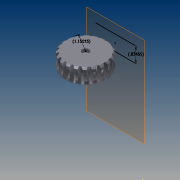
# Autodesk Inventor part: Worm Gear
Saved by Autodesk Inventor 2015 SP1 (Build 190203100, 203)
## iProperties
Created: 2015-04-26
Part Number: Worm Gear
Material: ABS Plastic
Document SubType Name: Modeling
Designer: Trevor
Categories: <?xml version="1.0" encoding="UTF-16"?> <MemberInstance><Categories><FamilyTemplate><FamilyTemplateParameter ValueType="xs:double" Id="1" ObjectReferenceKey="da_z" ObjectType="kUserParameterObject"/><FamilyTemplateParameter ValueType="xs:double" Id="2" ObjectReferenceKey="da_b" ObjectType="kUserParameterObject"/><FamilyTemplateParameter ValueType="xs:double" Id="3" ObjectReferenceKey="da_beta" ObjectType="kUserParameterObject"/><FamilyTemplateParameter ValueType="xs:double" Id="4" ObjectReferenceKey="da_m" ObjectType="kUserParameterObject"/><FamilyTemplateParameter ValueType="xs:double" Id="5" ObjectReferenceKey="da_alpha" ObjectType="kUserParameterObject"/><FamilyTemplateParameter ValueType="xs:double" Id="6" ObjectReferenceKey="da_da" ObjectType="kUserParameterObject"/><FamilyTemplateParameter ValueType="xs:double" Id="7" ObjectReferenceKey="da_aw" ObjectType="kUserParameterObject"/><FamilyTemplateParameter ValueType="xs:double" Id="8" ObjectReferenceKey="da_px" ObjectType="kUserParameterObject"/><FamilyTemplateParameter ValueType="xs:double" Id="9" ObjectReferenceKey="da_d" ObjectType="kUserParameterObject"/><FamilyTemplateParameter ValueType="xs:double" Id="10" ObjectReferenceKey="da_dae" ObjectType="kUserParameterObject"/><FamilyTemplateParameter ValueType="xs:double" Id="11" ObjectReferenceKey="da_fi" ObjectType="kUserParameterObject"/><FamilyTemplateParameter ValueType="xs:string" Id="12" ObjectReferenceKey="EAIAABAAAAAWFwAAAAAAAIAAAAAAAAAA" ObjectType="83910656" SubObjectId="SurfaceGeometry"/></FamilyTemplate><ParamToTemplateMap><ParamToTemplate CategoryParameter="//CategoryParameter[@InternalName='046C89C9-8512-4d59-83FE-43B91F4F132A']" TemplateParameter="1"/><ParamToTemplate CategoryParameter="//CategoryParameter[@InternalName='2552DF32-E462-4b46-AEBF-C6C7768E72AC']" TemplateParameter="2"/><ParamToTemplate CategoryParameter="//CategoryParameter[@InternalName='C9EE641D-15FC-4fae-A226-E94C4372FDD7']" TemplateParameter="3"/><ParamToTemplate><ParamToTemplate CategoryParameter="//CategoryParameter[@InternalName='00B6519A-459B-49c7-AD84-2E56D39A5744']" ConstantValue="0.000000"/></ParamToTemplate><ParamToTemplate><ParamToTemplate CategoryParameter="//CategoryParameter[@InternalName='04B31F0E-C7A6-4894-AA32-9629BEFACF47']" ConstantValue="1.000000"/></ParamToTemplate><ParamToTemplate><ParamToTemplate CategoryParameter="//CategoryParameter[@InternalName='43CBEC2E-7847-49e7-A936-2F7889FCB2D9']" ConstantValue="0.200000"/></ParamToTemplate><ParamToTemplate><ParamToTemplate CategoryParameter="//CategoryParameter[@InternalName='B1EFC894-105D-4ebd-86BF-FA20ED196853']" ConstantValue="0.300000"/></ParamToTemplate><ParamToTemplate><ParamToTemplate CategoryParameter="//CategoryParameter[@InternalName='51175063-3D10-4879-93E8-6246FE8B403D']" ConstantValue="2060110000.000000"/></ParamToTemplate><ParamToTemplate><ParamToTemplate CategoryParameter="//CategoryParameter[@InternalName='A3A52E27-4454-46a9-B0BD-C932399B70AF']" ConstantValue="0.300000"/></ParamToTemplate><ParamToTemplate CategoryParameter="//CategoryParameter[@InternalName='91B76062-C214-41d9-B1B9-14D2AB99603D']" TemplateParameter="4"/><ParamToTemplate CategoryParameter="//CategoryParameter[@InternalName='2D373A89-B862-43d6-8D0B-0CBF12AB9F6C']" TemplateParameter="5"/><ParamToTemplate CategoryParameter="//CategoryParameter[@InternalName='37777632-D6A2-4fac-9D53-DB8ACD95C989']" TemplateParameter="6"/><ParamToTemplate CategoryParameter="//CategoryParameter[@InternalName='FD1017F1-B727-4f7e-9707-0F86F1FF9423']" TemplateParameter="7"/><ParamToTemplate CategoryParameter="//CategoryParameter[@InternalName='3BF567DA-17EF-48d8-80EA-D119B07F6463']" TemplateParameter="8"/><ParamToTemplate CategoryParameter="//CategoryParameter[@InternalName='BF5A1E7E-5373-4a22-AAD3-F583781FCF3C']" TemplateParameter="9"/><ParamToTemplate CategoryParameter="//CategoryParameter[@InternalName='2A200944-5A8C-41ca-B96E-8520D2E510F1']" TemplateParameter="10"/><ParamToTemplate CategoryParameter="//CategoryParameter[@InternalName='E77AC4FD-7B43-4566-B0ED-7CA70B976BC8']" TemplateParameter="11"/><ParamToTemplate><ParamToTemplate CategoryParameter="//CategoryParameter[@InternalName='D4F72237-D604-435a-AD0B-F738B7463A00']" ConstantValue="110.000000"/></ParamToTemplate><ParamToTemplate><ParamToTemplate CategoryParameter="//CategoryParameter[@InternalName='9E1B4470-B2D3-4ff1-B813-535BB4CDF51A']" ConstantValue="1998100.000000"/></ParamToTemplate><ParamToTemplate><ParamToTemplate CategoryParameter="//CategoryParameter[@InternalName='A7A89E9A-52E6-4d4f-86CF-A81914F22AA4']" ConstantValue="250000000.000000"/></ParamToTemplate><ParamToTemplate><ParamToTemplate CategoryParameter="//CategoryParameter[@InternalName='B02FABAC-469F-4ad8-A219-DB4578299DF6']" ConstantValue="250000000.000000"/></ParamToTemplate><ParamToTemplate><ParamToTemplate CategoryParameter="//CategoryParameter[@InternalName='E6981962-40D5-4343-A0AD-C263FCC47E10']" ConstantValue="9.000000"/></ParamToTemplate><ParamToTemplate><ParamToTemplate CategoryParameter="//CategoryParameter[@InternalName='B958E99F-2BCD-4955-8634-793EB7B37B89']" ConstantValue="8.000000"/></ParamToTemplate><ParamToTemplate><ParamToTemplate CategoryParameter="//CategoryParameter[@InternalName='4AD49A87-569D-440f-A541-E3B52A6A9DCE']" ConstantValue="1219.200000"/></ParamToTemplate><ParamToTemplate><ParamToTemplate CategoryParameter="//CategoryParameter[@InternalName='4E5813A0-330D-4b41-BE23-D880B01A1D55']" ConstantValue="1653600.000000"/></ParamToTemplate><ParamToTemplate><ParamToTemplate CategoryParameter="//CategoryParameter[@InternalName='19EB8C86-AA88-4253-B4AA-2F5DF1CE171A']" ConstantValue="5512.000000"/></ParamToTemplate><ParamToTemplate CategoryParameter="//CategoryParameter[@InternalName='27C3BAF2-7550-4e4b-AE2C-0DB134B7D9B7']" TemplateParameter="12"/></ParamToTemplateMap><Category DisplayName="Gear" InternalName="DC85795E-93AB-48d5-8EEE-5A27447B64BD" Mnemonic="Gear"><CategoryParameter DisplayName="z" InternalName="046C89C9-8512-4d59-83FE-43B91F4F132A" Mnemonic="z"/><CategoryParameter DisplayName="b|.2|" InternalName="2552DF32-E462-4b46-AEBF-C6C7768E72AC" Mnemonic="b"/><CategoryParameter DisplayName="||b|" InternalName="C9EE641D-15FC-4fae-A226-E94C4372FDD7" Mnemonic="beta"/><CategoryParameter DisplayName="x" InternalName="00B6519A-459B-49c7-AD84-2E56D39A5744" Mnemonic="x"/><CategoryParameter DisplayName="a*" InternalName="04B31F0E-C7A6-4894-AA32-9629BEFACF47" Mnemonic="a"/><CategoryParameter DisplayName="c*" InternalName="43CBEC2E-7847-49e7-A936-2F7889FCB2D9" Mnemonic="c"/><CategoryParameter DisplayName="r|.f|*" InternalName="B1EFC894-105D-4ebd-86BF-FA20ED196853" Mnemonic="rf"/><CategoryParameter DisplayName="E" InternalName="51175063-3D10-4879-93E8-6246FE8B403D" Mnemonic="E"/><CategoryParameter DisplayName="||m|" InternalName="A3A52E27-4454-46a9-B0BD-C932399B70AF" Mnemonic="mi"/><Category DisplayName="WormGear" InternalName="1B25C7EF-093B-4025-B3D3-619CD2A4550C" Mnemonic="WormGear"><CategoryParameter DisplayName="m" InternalName="91B76062-C214-41d9-B1B9-14D2AB99603D" Mnemonic="m"/><CategoryParameter DisplayName="||a|" InternalName="2D373A89-B862-43d6-8D0B-0CBF12AB9F6C" Mnemonic="alpha"/><CategoryParameter DisplayName="d|.a|" InternalName="37777632-D6A2-4fac-9D53-DB8ACD95C989" Mnemonic="da"/><CategoryParameter DisplayName="a|.w|" InternalName="FD1017F1-B727-4f7e-9707-0F86F1FF9423" Mnemonic="aw"/><CategoryParameter DisplayName="p|.x|" InternalName="3BF567DA-17EF-48d8-80EA-D119B07F6463" Mnemonic="px"/><CategoryParameter DisplayName="d" InternalName="BF5A1E7E-5373-4a22-AAD3-F583781FCF3C" Mnemonic="d"/><CategoryParameter DisplayName="dae" InternalName="2A200944-5A8C-41ca-B96E-8520D2E510F1" Mnemonic="dae"/><CategoryParameter DisplayName="||d|" InternalName="E77AC4FD-7B43-4566-B0ED-7CA70B976BC8" Mnemonic="fi"/><CategoryParameter DisplayName="VHV" InternalName="D4F72237-D604-435a-AD0B-F738B7463A00" Mnemonic="VHV"/><CategoryParameter DisplayName="||s||.Hlim|" InternalName="9E1B4470-B2D3-4ff1-B813-535BB4CDF51A" Mnemonic="sHlim"/><CategoryParameter DisplayName="N|.Flim|" InternalName="A7A89E9A-52E6-4d4f-86CF-A81914F22AA4" Mnemonic="NFlim"/><CategoryParameter DisplayName="N|.Hlim|" InternalName="B02FABAC-469F-4ad8-A219-DB4578299DF6" Mnemonic="NHlim"/><CategoryParameter DisplayName="q|.F|" InternalName="E6981962-40D5-4343-A0AD-C263FCC47E10" Mnemonic="qF"/><CategoryParameter DisplayName="q|.H|" InternalName="B958E99F-2BCD-4955-8634-793EB7B37B89" Mnemonic="qH"/><CategoryParameter DisplayName="v|.max|" InternalName="4AD49A87-569D-440f-A541-E3B52A6A9DCE" Mnemonic="maxv"/><CategoryParameter DisplayName="S|.n|" InternalName="4E5813A0-330D-4b41-BE23-D880B01A1D55" Mnemonic="Sn"/><CategoryParameter DisplayName="K|.w|" InternalName="19EB8C86-AA88-4253-B4AA-2F5DF1CE171A" Mnemonic="Kw"/><CategoryParameter DisplayName="PitchDiameter" InternalName="27C3BAF2-7550-4e4b-AE2C-0DB134B7D9B7" Mnemonic="IDS_PITCHDIAM"/></Category></Category></Categories></MemberInstance>
Density: 1.06 g/cm^3
Appearance: Smooth - White
CustomPartVersion: 1
r_gear: 1.15015 in
w_gear: 0.83465 in
Author: Trevor
Autodesk Inventor part; units mm, degrees
ref_plane "YZ Plane" through (0, 0, 0) normal (1, 0, 0) x (0, 1, 0)
ref_plane "XZ Plane" through (0, 0, 0) normal (0, 1, 0) x (-1, 0, 0)
ref_plane "XY Plane" through (0, 0, 0) normal (0, 0, 1) x (1, 0, 0)
ref_plane "Tooth Plane" through (0, -10, 0) normal (-0.0995037, 0, 0.9950372) x (0, 1, 0)
sketch "Base Body Sketch" plane through (0, 0, 0) normal (1, 0, 0) x (0, 1, 0)
  line L0 (0, -22.6382) -> (0, 22.6382) projected
  line L1 (0, 10.6) -> (27.1524, 10.6)
  line L2 (27.1524, 10.6) -> (29.2138, 8.605)
  line L3 (-10.9148, 0) -> (65.4891, 0) construction
  circle A0 centre (38.1049, 0) radius 10.1613
  line L4 (29.2138, 8.605) -> (29.2138, -8.605)
  line L5 (0, -10.6) -> (27.1524, -10.6)
  line L6 (0, 10.6) -> (0, -10.6)
  line L7 (27.1524, -10.6) -> (29.2138, -8.605)
  dimension "d50" = 44.063
  dimension "d87" = 58.4276
  dimension "d89" = 20.3226
  dimension "d92" = 21.2
  dimension "d93" = 38.1049
  constraints: 14 end point, 3 symmetric about line, 2 perpendicular, 2 point on line, 1 centre point, 1 collinear
  measures "d50" angle of L2 L1
  measures "d87" diameter of L4 L0
  measures "d89" diameter of A0
  measures "d92" distance of L1.start L5.start
  measures "d93" distance from line of A0.centre L6
revolve "Base Body" add sketch "Base Body Sketch" angle 360 about axis through (0, 0, 0) along (0, 0, 1) picked at (28.9449, 1.0114) contours L0 L1 L2 L4 A0 L7 L5 | A0 L4
revolve "Base Body2" cut sketch "Base Body Sketch" angle 360 about axis through (0, 0, 0) along (0, 0, 1) contours L4 A0 | A0 L4
sketch "Tooth Sketch" plane through (0, -10, 0) normal (-0.0995037, 0, 0.9950372) x (0, 1, 0)
  line L0 (10, 4.1701) -> (10, -5.5057) projected
  line L1 (-36.0849, 0) -> (17.6808, 0) projected
  line L2 (-28.1049, 3.5037) -> (-28.1049, -3.5037)
  line L3 (-28.1049, -3.5037) -> (-18.4517, -3.5037)
  line L4 (-18.4517, -3.5037) -> (-12.3549, -1.2847)
  line L5 (-12.3549, -1.2847) -> (-12.3549, 0)
  line L6 (-12.3549, 1.2847) -> (-18.4517, 3.5037)
  line L7 (-18.4517, 3.5037) -> (-28.1049, 3.5037)
  line L8 (-12.3549, 1.2847) -> (-12.3549, 0)
  line L9 (-15.4033, 0) -> (-15.4033, -2.3942) construction
  dimension "d38" = 38.1049
  dimension "d39" = 20
  dimension "d40" = 9.6532
  dimension "d41" = 12.7017
  dimension "d42" = 2.3942
  constraints: 16 end point, 4 perpendicular, 3 equal length, 2 point on line, 1 midpoint, 1 parallel, 1 vertical
  measures "d38" distance between parallel lines of L0 L2
  measures "d39" angle of L6 L7
  measures "d40" distance of L6.end L2.start
  measures "d41" distance between parallel lines of L2 L9
  measures "d42" distance of L9.start L9.end
sketch "Sketch8" plane through (0, 0, 10.6) normal (0, 0, 1) x (1, 0, 0)
  circle A0 centre (0, 0) radius 27.1524 projected
  circle A1 centre (0, 0) radius 25.4033
  dimension "d77" = 50.8066
  constraints: 1 centre point, 1 coincident
  measures "d77" diameter of A1
surface extrude "Pitch Diameter" sketch "Sketch8" against normal blind 21.2 shown no curves A1
ref_plane "Work Plane13" through (0, 0, 0) normal (-0.1564345, 0.9876883, 0) x (0, 0, 1)
revolve "Tooth" cut sketch "Tooth Sketch" angle 360 about axis through (-3.4863, -38.1049, -0.3486) along (0.9950372, 0, 0.0995037)
pattern_circular "Tooth Pattern" count 20 over 360 about axis through (0, 0, 0) along (0, 0, 1) of "Tooth"
ref_plane "Work Plane14" through (0, 0, 0) normal (0.9876883, 0.1564345, 0) x (0, 0, 1)
ref_plane "Work Plane15" through (0, 0, 0) normal (0, -1, 0) x (0, 0, 1)
sketch "Sketch9" plane through (0, 0, 10.6) normal (0, 0, 1) x (0.9811818, -0.1930863, 0)
  point P0 (0, 0)
sketch "Sketch10" plane through (0, 0, 10.6) normal (0, 0, 1) x (0.9811818, -0.1930863, 0)
  arc A0 (-27.1775, 10.7158) -> (-28.4317, 6.7143) centre (0, 0) ccw projected
  dimension "r_gear" = 29.2138
  measures "r_gear" radius of A0
sketch "Sketch11" plane through (0, 0, -10.6) normal (0, 0, -1) x (-0.907286, 0.4205141, 0)
  line L0 (-3.3676, 3.3676) -> (3.3676, 3.3676)
  line L1 (3.3676, 3.3676) -> (3.3676, -3.3676)
  line L2 (3.3676, -3.3676) -> (-3.3676, -3.3676)
  line L3 (-3.3676, -3.3676) -> (-3.3676, 3.3676)
  line L4 (-3.3676, 3.3676) -> (3.3676, -3.3676) construction
  line L5 (3.3676, 3.3676) -> (-3.3676, -3.3676) construction
  circle A0 centre (0, 0) radius 4.7625
  dimension "d95" = 6.7352
  constraints: 12 end point, 2 midpoint, 2 parallel, 2 perpendicular, 1 coincident, 1 horizontal, 3 other
  measures "d95" distance of L0.end L1.end
extrude "Extrusion1" add sketch "Sketch11" along normal blind 4.7625
sketch "Sketch12" plane through (0, 0, -15.3625) normal (0, 0, -1) x (-1, 0, 0)
  circle A0 centre (0, 0) radius 4.7625 projected
  line L0 (-3.3676, 3.3676) -> (3.3676, 3.3676)
  line L1 (3.3676, 3.3676) -> (3.3676, -3.3676)
  line L2 (3.3676, -3.3676) -> (-3.3676, -3.3676)
  line L3 (-3.3676, -3.3676) -> (-3.3676, 3.3676)
  line L4 (-3.3676, 3.3676) -> (3.3676, -3.3676) construction
  line L5 (3.3676, 3.3676) -> (-3.3676, -3.3676) construction
  constraints: 12 end point, 2 midpoint, 2 parallel, 2 perpendicular, 1 horizontal, 2 other
extrude "Extrusion2" add sketch "Sketch12" along normal blind 6.35 contours L1 L2 L3 L0
ref_plane "Work Plane16" through (0, 41.4619, -39.2906) normal (0, -1, 0) x (1, 0, 0)
sketch "Sketch13" plane through (0, 0, 10.6) normal (0, 0, 1) x (0.9811818, -0.1930863, 0)
  circle A0 centre (0, 0) radius 4.7625 projected
extrude "Extrusion3" cut sketch "Sketch13" against normal blind 4.7625
sketch "Sketch14" plane through (0, 41.4619, -39.2906) normal (0, -1, 0) x (1, 0, 0)
  line L0 (-4.7625, 49.8906) -> (4.7625, 49.8906) projected
  line L1 (-10.6945, 49.8906) -> (-10.4631, 49.8906) projected
  line L2 (-10.4631, 49.8906) -> (-7.9344, 49.8906) projected
  line L3 (-7.9344, 49.8906) -> (-7.9706, 49.8906) projected
  line L4 (-2.4587, 49.8906) -> (-7.9706, 49.8906) projected
  line L5 (-2.4587, 49.8906) -> (-2.3511, 49.8906) projected
  line L6 (-2.3511, 49.8906) -> (0.2311, 49.8906) projected
  line L7 (0.2311, 49.8906) -> (0.4405, 49.8906) projected
  line L8 (6.0177, 49.8906) -> (0.4405, 49.8906) projected
  line L9 (6.0177, 49.8906) -> (5.9911, 49.8906) projected
  line L10 (5.9911, 49.8906) -> (8.3739, 49.8906) projected
  line L11 (8.3739, 49.8906) -> (8.8084, 49.8906) projected
  line L12 (13.9051, 49.8906) -> (8.8084, 49.8906) projected
  line L13 (13.9051, 49.8906) -> (13.7468, 49.8906) projected
  line L14 (13.7468, 49.8906) -> (15.6971, 49.8906) projected
  line L15 (15.6971, 49.8906) -> (16.314, 49.8906) projected
  line L16 (20.4313, 49.8906) -> (16.314, 49.8906) projected
  line L17 (20.4313, 49.8906) -> (20.1568, 49.8906) projected
  line L18 (20.1568, 49.8906) -> (21.4837, 49.8906) projected
  line L19 (21.4837, 49.8906) -> (22.2228, 49.8906) projected
  line L20 (24.9576, 49.8906) -> (22.2228, 49.8906) projected
  line L21 (24.9576, 49.8906) -> (24.5938, 49.8906) projected
  line L22 (24.5938, 49.8906) -> (25.1673, 49.8906) projected
  line L23 (25.1673, 49.8906) -> (25.9562, 49.8906) projected
  line L24 (27.0409, 49.8906) -> (25.9562, 49.8906) projected
  line L25 (27.0409, 49.8906) -> (26.6234, 49.8906) projected
  line L26 (26.6234, 49.8906) -> (26.3874, 49.8906) projected
  line L27 (26.3874, 49.8906) -> (27.1488, 49.8906) projected
  line L28 (26.4772, 49.8906) -> (27.1488, 49.8906) projected
  line L29 (26.4772, 49.8906) -> (26.0468, 49.8906) projected
  line L30 (26.0468, 49.8906) -> (25.0245, 49.8906) projected
  line L31 (25.0245, 49.8906) -> (25.684, 49.8906) projected
  line L32 (23.3217, 49.8906) -> (25.684, 49.8906) projected
  line L33 (23.3217, 49.8906) -> (22.9207, 49.8906) projected
  line L34 (22.9207, 49.8906) -> (21.212, 49.8906) projected
  line L35 (21.212, 49.8906) -> (21.705, 49.8906) projected
  line L36 (17.8834, 49.8906) -> (21.705, 49.8906) projected
  line L37 (17.8834, 49.8906) -> (17.5509, 49.8906) projected
  line L38 (17.5509, 49.8906) -> (15.3232, 49.8906) projected
  line L39 (15.3232, 49.8906) -> (15.6013, 49.8906) projected
  line L40 (10.6945, 49.8906) -> (15.6013, 49.8906) projected
  line L41 (10.6945, 49.8906) -> (10.4631, 49.8906) projected
  line L42 (10.4631, 49.8906) -> (7.9344, 49.8906) projected
  line L43 (7.9344, 49.8906) -> (7.9706, 49.8906) projected
  line L44 (2.4587, 49.8906) -> (7.9706, 49.8906) projected
  line L45 (2.4587, 49.8906) -> (2.3511, 49.8906) projected
  line L46 (2.3511, 49.8906) -> (-0.2311, 49.8906) projected
  line L47 (-0.2311, 49.8906) -> (-0.4405, 49.8906) projected
  line L48 (-6.0177, 49.8906) -> (-0.4405, 49.8906) projected
  line L49 (-6.0177, 49.8906) -> (-5.9911, 49.8906) projected
  line L50 (-5.9911, 49.8906) -> (-8.3739, 49.8906) projected
  line L51 (-8.3739, 49.8906) -> (-8.8084, 49.8906) projected
  line L52 (-13.9051, 49.8906) -> (-8.8084, 49.8906) projected
  line L53 (-13.9051, 49.8906) -> (-13.7468, 49.8906) projected
  line L54 (-13.7468, 49.8906) -> (-15.6971, 49.8906) projected
  line L55 (-15.6971, 49.8906) -> (-16.314, 49.8906) projected
  line L56 (-20.4313, 49.8906) -> (-16.314, 49.8906) projected
  line L57 (-20.4313, 49.8906) -> (-20.1568, 49.8906) projected
  line L58 (-20.1568, 49.8906) -> (-21.4837, 49.8906) projected
  line L59 (-21.4837, 49.8906) -> (-22.2228, 49.8906) projected
  line L60 (-24.9576, 49.8906) -> (-22.2228, 49.8906) projected
  line L61 (-24.9576, 49.8906) -> (-24.5938, 49.8906) projected
  line L62 (-24.5938, 49.8906) -> (-25.1673, 49.8906) projected
  line L63 (-25.1673, 49.8906) -> (-25.9562, 49.8906) projected
  line L64 (-27.0409, 49.8906) -> (-25.9562, 49.8906) projected
  line L65 (-27.0409, 49.8906) -> (-26.6234, 49.8906) projected
  line L66 (-26.6234, 49.8906) -> (-26.3874, 49.8906) projected
  line L67 (-26.3874, 49.8906) -> (-27.1488, 49.8906) projected
  line L68 (-26.4772, 49.8906) -> (-27.1488, 49.8906) projected
  line L69 (-26.4772, 49.8906) -> (-26.0468, 49.8906) projected
  line L70 (-26.0468, 49.8906) -> (-25.0245, 49.8906) projected
  line L71 (-25.0245, 49.8906) -> (-25.684, 49.8906) projected
  line L72 (-23.3217, 49.8906) -> (-25.684, 49.8906) projected
  line L73 (-23.3217, 49.8906) -> (-22.9207, 49.8906) projected
  line L74 (-22.9207, 49.8906) -> (-21.212, 49.8906) projected
  line L75 (-21.212, 49.8906) -> (-21.705, 49.8906) projected
  line L76 (-17.8834, 49.8906) -> (-21.705, 49.8906) projected
  line L77 (-17.8834, 49.8906) -> (-17.5509, 49.8906) projected
  line L78 (-17.5509, 49.8906) -> (-15.3232, 49.8906) projected
  line L79 (-15.3232, 49.8906) -> (-15.6013, 49.8906) projected
  line L80 (-10.6945, 49.8906) -> (-15.6013, 49.8906) projected
  line L81 (4.7625, 28.6906) -> (-4.7625, 28.6906) projected
  line L82 (-8.3739, 28.6906) -> (-8.8084, 28.6906) projected
  line L83 (-8.8084, 28.6906) -> (-13.9051, 28.6906) projected
  line L84 (-13.9051, 28.6906) -> (-13.7468, 28.6906) projected
  line L85 (-13.7468, 28.6906) -> (-15.6971, 28.6906) projected
  line L86 (-15.6971, 28.6906) -> (-16.314, 28.6906) projected
  line L87 (-16.314, 28.6906) -> (-20.4313, 28.6906) projected
  line L88 (-20.4313, 28.6906) -> (-20.1568, 28.6906) projected
  line L89 (-20.1568, 28.6906) -> (-21.4837, 28.6906) projected
  line L90 (-21.4837, 28.6906) -> (-22.2228, 28.6906) projected
  line L91 (-22.2228, 28.6906) -> (-24.9576, 28.6906) projected
  line L92 (-24.9576, 28.6906) -> (-24.5938, 28.6906) projected
  line L93 (-24.5938, 28.6906) -> (-25.1673, 28.6906) projected
  line L94 (-25.1673, 28.6906) -> (-25.9562, 28.6906) projected
  line L95 (-25.9562, 28.6906) -> (-27.0409, 28.6906) projected
  line L96 (-27.0409, 28.6906) -> (-26.6234, 28.6906) projected
  line L97 (-26.6234, 28.6906) -> (-26.3874, 28.6906) projected
  line L98 (-26.3874, 28.6906) -> (-27.1488, 28.6906) projected
  line L99 (-27.1488, 28.6906) -> (-26.4772, 28.6906) projected
  line L100 (-26.4772, 28.6906) -> (-26.0468, 28.6906) projected
  line L101 (-26.0468, 28.6906) -> (-25.0245, 28.6906) projected
  line L102 (-25.0245, 28.6906) -> (-25.684, 28.6906) projected
  line L103 (-25.684, 28.6906) -> (-23.3217, 28.6906) projected
  line L104 (-23.3217, 28.6906) -> (-22.9207, 28.6906) projected
  line L105 (-22.9207, 28.6906) -> (-21.212, 28.6906) projected
  line L106 (-21.212, 28.6906) -> (-21.705, 28.6906) projected
  line L107 (-21.705, 28.6906) -> (-17.8834, 28.6906) projected
  line L108 (-17.8834, 28.6906) -> (-17.5509, 28.6906) projected
  line L109 (-17.5509, 28.6906) -> (-15.3232, 28.6906) projected
  line L110 (-15.3232, 28.6906) -> (-15.6013, 28.6906) projected
  line L111 (-15.6013, 28.6906) -> (-10.6945, 28.6906) projected
  line L112 (-10.6945, 28.6906) -> (-10.4631, 28.6906) projected
  line L113 (-10.4631, 28.6906) -> (-7.9344, 28.6906) projected
  line L114 (-7.9344, 28.6906) -> (-7.9706, 28.6906) projected
  line L115 (-7.9706, 28.6906) -> (-2.4587, 28.6906) projected
  line L116 (-2.4587, 28.6906) -> (-2.3511, 28.6906) projected
  line L117 (-2.3511, 28.6906) -> (0.2311, 28.6906) projected
  line L118 (0.2311, 28.6906) -> (0.4405, 28.6906) projected
  line L119 (0.4405, 28.6906) -> (6.0177, 28.6906) projected
  line L120 (6.0177, 28.6906) -> (5.9911, 28.6906) projected
  line L121 (5.9911, 28.6906) -> (8.3739, 28.6906) projected
  line L122 (8.3739, 28.6906) -> (8.8084, 28.6906) projected
  line L123 (8.8084, 28.6906) -> (13.9051, 28.6906) projected
  line L124 (13.9051, 28.6906) -> (13.7468, 28.6906) projected
  line L125 (13.7468, 28.6906) -> (15.6971, 28.6906) projected
  line L126 (15.6971, 28.6906) -> (16.314, 28.6906) projected
  line L127 (16.314, 28.6906) -> (20.4313, 28.6906) projected
  line L128 (20.4313, 28.6906) -> (20.1568, 28.6906) projected
  line L129 (20.1568, 28.6906) -> (21.4837, 28.6906) projected
  line L130 (21.4837, 28.6906) -> (22.2228, 28.6906) projected
  line L131 (22.2228, 28.6906) -> (24.9576, 28.6906) projected
  line L132 (24.9576, 28.6906) -> (24.5938, 28.6906) projected
  line L133 (24.5938, 28.6906) -> (25.1673, 28.6906) projected
  line L134 (25.1673, 28.6906) -> (25.9562, 28.6906) projected
  line L135 (25.9562, 28.6906) -> (27.0409, 28.6906) projected
  line L136 (27.0409, 28.6906) -> (26.6234, 28.6906) projected
  line L137 (26.6234, 28.6906) -> (26.3874, 28.6906) projected
  line L138 (26.3874, 28.6906) -> (27.1488, 28.6906) projected
  line L139 (27.1488, 28.6906) -> (26.4772, 28.6906) projected
  line L140 (26.4772, 28.6906) -> (26.0468, 28.6906) projected
  line L141 (26.0468, 28.6906) -> (25.0245, 28.6906) projected
  line L142 (25.0245, 28.6906) -> (25.684, 28.6906) projected
  line L143 (25.684, 28.6906) -> (23.3217, 28.6906) projected
  line L144 (23.3217, 28.6906) -> (22.9207, 28.6906) projected
  line L145 (22.9207, 28.6906) -> (21.212, 28.6906) projected
  line L146 (21.212, 28.6906) -> (21.705, 28.6906) projected
  line L147 (21.705, 28.6906) -> (17.8834, 28.6906) projected
  line L148 (17.8834, 28.6906) -> (17.5509, 28.6906) projected
  line L149 (17.5509, 28.6906) -> (15.3232, 28.6906) projected
  line L150 (15.3232, 28.6906) -> (15.6013, 28.6906) projected
  line L151 (15.6013, 28.6906) -> (10.6945, 28.6906) projected
  line L152 (10.6945, 28.6906) -> (10.4631, 28.6906) projected
  line L153 (10.4631, 28.6906) -> (7.9344, 28.6906) projected
  line L154 (7.9344, 28.6906) -> (7.9706, 28.6906) projected
  line L155 (7.9706, 28.6906) -> (2.4587, 28.6906) projected
  line L156 (2.4587, 28.6906) -> (2.3511, 28.6906) projected
  line L157 (2.3511, 28.6906) -> (-0.2311, 28.6906) projected
  line L158 (-0.2311, 28.6906) -> (-0.4405, 28.6906) projected
  line L159 (-0.4405, 28.6906) -> (-6.0177, 28.6906) projected
  line L160 (-6.0177, 28.6906) -> (-5.9911, 28.6906) projected
  line L161 (-5.9911, 28.6906) -> (-8.3739, 28.6906) projected
  point P0 (0, 39.2906)
  dimension "w_gear" = 21.2
  measures "w_gear" distance of L138.end L27.end
hole "Hole3" at (0, 0, 10.6) direction (0, 0, -1) diameter 2.81 depth 6.35
equation "\"d50\" = da_fi"
equation "\"d87\" = da_dae"
equation "\"d89\" = 2 * da_aw - da_da"
equation "\"d92\" = da_b"
equation "\"d93\" = da_aw"
equation "\"d95\" = l_key"
equation "\"d96\" = t"
equation "\"d98\" = d_key"
equation "\"d100\" = t"
equation "\"d38\" = da_aw"
equation "\"d39\" = da_alfat"
equation "\"d40\" = 0.5 * da_df1"
equation "\"d41\" = 0.5 * da_d1"
equation "\"d42\" = 0.3 * da_px"
equation "\"d77\" = da_dw"
equation "\"d78\" = da_b"
equation "\"da_aw\" = 38.10494"
equation "\"da_fi\" = 44.0629deg"
equation "\"da_b\" = 21.2"
equation "\"da_df\" = 44.7098"
equation "\"da_da\" = 55.88725"
equation "\"da_beta\" = 5.710593deg"
equation "\"da_alfat\" = 20deg"
equation "\"da_df1\" = 19.3065"
equation "\"da_da1\" = 30.48395"
equation "\"da_d1\" = 25.40329"
equation "\"da_px\" = 7.98068"
equation "\"d68\" = da_aw"
equation "\"da_dw\" = 50.80659"
equation "\"da_rightdir\" = 0"
equation "\"d86\" = da_aw"
equation "\"da_dae\" = 58.42757"
equation "\"l_key\" = 6.735192"
equation "\"t\" = 4.7625"
equation "\"d_key\" = 6.35"
body "Solid1"
body "Srf1"
